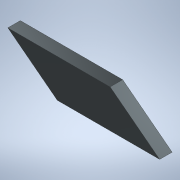
# Autodesk Inventor part: Brazo_C
Saved by Autodesk Inventor 2020 (Build 240168000, 168)
## iProperties
Created: 2020-07-18
Part Number: Brazo_C
Material: Hierro, fundido
Document SubType Name: Modeling
Designer: louis
Density: 7.15 g/cm^3
Appearance: Gris hierro
Author: louis
Autodesk Inventor part; units mm, degrees
ref_plane "YZ Plane" through (0, 0, 0) normal (1, 0, 0) x (0, 1, 0)
ref_plane "XZ Plane" through (0, 0, 0) normal (0, 1, 0) x (-1, 0, 0)
ref_plane "XY Plane" through (0, 0, 0) normal (0, 0, 1) x (1, 0, 0)
sketch "Boceto1" plane through (0, 0, 0) normal (0, 0, 1) x (1, 0, 0)
  line L0 (-75.5202, 28.6978) -> (6.4858, 28.6978)
  line L1 (46.1178, -1.7877) -> (-35.8882, -1.7877)
  line L2 (-75.5202, 28.6978) -> (-35.8882, -1.7877)
  line L3 (-35.8882, -1.7877) -> (-35.8882, -1.7877)
  line L4 (6.4858, 28.6978) -> (31.8808, 9.1636)
  line L5 (31.8808, 9.1636) -> (46.1178, -1.7877)
  line L6 (-35.8882, -1.7877) -> (-20.031, -13.9853)
  point P0 (0, 0)
  point P1 (-35.8882, -1.7877)
  dimension "d3" = 82.006
  dimension "d13" = 37.568
  dimension "d14" = 37.568
  dimension "d15" = 30.4855
  constraints: 14 end point, 2 horizontal, 1 parallel, 1 point on line
  measures "d3" distance of L1.start L1.end
  measures "d13" angle of L0 L2
  measures "d14" angle of L1 L4
  measures "d15" distance between parallel lines of L1 L0
extrude "Extrusión1" add sketch "Boceto1" along normal blind 10
